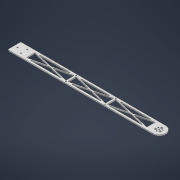
# Autodesk Inventor part: Top_Arm
Saved by Autodesk Inventor 2022 (Build 260153000, 153)
## iProperties
Created: 2023-02-15
Part Number: Top_Arm
Material: Generic
Document SubType Name: Modeling
Designer: dzw04
Density: 1 g/cm^3
Appearance: Default
Author: dzw04
Autodesk Inventor part; units mm, degrees
ref_plane "YZ Plane" through (0, 0, 0) normal (1, 0, 0) x (0, 1, 0)
ref_plane "XZ Plane" through (0, 0, 0) normal (0, 1, 0) x (-1, 0, 0)
ref_plane "XY Plane" through (0, 0, 0) normal (0, 0, 1) x (1, 0, 0)
sketch "Sketch1" plane through (0, 0, 0) normal (0, 1, 0) x (-1, 0, 0)
  arc A0 (74.0881, -0.9737) -> (74.0881, 0.9737) centre (73.8602, 0) ccw
  line L0 (74.0881, 0.9737) -> (26.2278, 12.1722)
  arc A1 (26.2278, 12.1722) -> (25, 11.1985) centre (26, 11.1985) ccw
  line L1 (25, 11.1985) -> (25, -11.1985)
  arc A2 (25, -11.1985) -> (26.2278, -12.1722) centre (26, -11.1985) ccw
  line L2 (26.2278, -12.1722) -> (74.0881, -0.9737)
  circle A3 centre (410, -10) radius 1.5
  line L3 (250.0605, -12.029) -> (212.2835, -2.7232)
  arc A4 (212.2835, -2.7232) -> (202.7161, -2.7232) centre (207.4998, -22.1427) ccw
  line L4 (202.7161, -2.7232) -> (164.9392, -12.029)
  arc A5 (164.9392, -12.029) -> (165.1783, -14) centre (165.1783, -13) ccw
  line L5 (165.1783, -14) -> (249.8213, -14)
  arc A6 (249.8213, -14) -> (250.0605, -12.029) centre (249.8213, -13) ccw
  line L6 (212.2835, 2.7232) -> (250.0605, 12.029)
  arc A7 (250.0605, 12.029) -> (249.8213, 14) centre (249.8213, 13) ccw
  line L7 (249.8213, 14) -> (165.1783, 14)
  arc A8 (165.1783, 14) -> (164.9392, 12.029) centre (165.1783, 13) ccw
  line L8 (164.9392, 12.029) -> (202.7161, 2.7232)
  arc A9 (202.7161, 2.7232) -> (212.2835, 2.7232) centre (207.4998, 22.1427) ccw
  circle A10 centre (6.4952, -3.75) radius 1.5
  line L9 (80.2767, -2.6067) -> (40.0191, -12.0263)
  arc A11 (40.0191, -12.0263) -> (40.2469, -14) centre (40.2469, -13) ccw
  line L10 (40.2469, -14) -> (129.4198, -14)
  arc A12 (129.4198, -14) -> (129.6476, -12.0263) centre (129.4198, -13) ccw
  line L11 (129.6476, -12.0263) -> (89.3899, -2.6067)
  arc A13 (89.3899, -2.6067) -> (80.2767, -2.6067) centre (84.8333, -22.0807) ccw
  line L12 (374.9809, -12.0263) -> (334.7231, -2.6067)
  arc A14 (334.7231, -2.6067) -> (325.6099, -2.6067) centre (330.1665, -22.0807) ccw
  line L13 (325.6099, -2.6067) -> (285.3521, -12.0263)
  arc A15 (285.3521, -12.0263) -> (285.58, -14) centre (285.58, -13) ccw
  line L14 (285.58, -14) -> (374.753, -14)
  arc A16 (374.753, -14) -> (374.9809, -12.0263) centre (374.753, -13) ccw
  line L15 (150.6667, 11.1789) -> (150.6667, -11.1789)
  arc A17 (150.6667, -11.1789) -> (151.9059, -12.1499) centre (151.6667, -11.1789) ccw
  line L16 (151.9059, -12.1499) -> (197.2869, -0.971)
  arc A18 (197.2869, -0.971) -> (197.2869, 0.971) centre (197.0477, 0) ccw
  line L17 (197.2869, 0.971) -> (151.9059, 12.1499)
  arc A19 (151.9059, 12.1499) -> (150.6667, 11.1789) centre (151.6667, 11.1789) ccw
  circle A20 centre (0, 0) radius 1.5
  circle A21 centre (6.4952, 3.75) radius 2.75
  line L18 (89.3899, 2.6067) -> (138.0828, 14)
  line L19 (138.0828, 14) -> (40.2469, 14)
  arc A22 (40.2469, 14) -> (40.0191, 12.0263) centre (40.2469, 13) ccw
  line L20 (40.0191, 12.0263) -> (80.2767, 2.6067)
  arc A23 (80.2767, 2.6067) -> (89.3899, 2.6067) centre (84.8333, 22.0807) ccw
  arc A24 (388.7722, -12.1722) -> (390, -11.1985) centre (389, -11.1985) ccw
  line L21 (390, -11.1985) -> (390, 11.1985)
  arc A25 (390, 11.1985) -> (388.7722, 12.1722) centre (389, 11.1985) ccw
  line L22 (388.7722, 12.1722) -> (340.9118, 0.9737)
  arc A26 (340.9118, 0.9737) -> (340.9118, -0.9737) centre (341.1396, 0) ccw
  line L23 (340.9118, -0.9737) -> (388.7722, -12.1722)
  line L24 (334.7231, 2.6067) -> (374.9809, 12.0263)
  arc A27 (374.9809, 12.0263) -> (374.753, 14) centre (374.753, 13) ccw
  line L25 (374.753, 14) -> (285.58, 14)
  arc A28 (285.58, 14) -> (285.3521, 12.0263) centre (285.58, 13) ccw
  line L26 (285.3521, 12.0263) -> (325.6099, 2.6067)
  arc A29 (325.6099, 2.6067) -> (334.7231, 2.6067) centre (330.1665, 22.0807) ccw
  circle A30 centre (430, 0) radius 1.5
  circle A31 centre (0, -7.5) radius 2.75
  circle A32 centre (0, 7.5) radius 1.5
  line L27 (144.6667, -11.1985) -> (144.6667, 11.1985)
  arc A33 (144.6667, 11.1985) -> (143.4388, 12.1722) centre (143.6667, 11.1985) ccw
  line L28 (143.4388, 12.1722) -> (95.5786, 0.9737)
  arc A34 (95.5786, 0.9737) -> (95.5786, -0.9737) centre (95.8064, 0) ccw
  line L29 (95.5786, -0.9737) -> (143.4388, -12.1722)
  arc A35 (143.4388, -12.1722) -> (144.6667, -11.1985) centre (143.6667, -11.1985) ccw
  arc A36 (264.333, 11.1789) -> (263.0938, 12.1499) centre (263.333, 11.1789) ccw
  line L30 (263.0938, 12.1499) -> (217.7128, 0.971)
  arc A37 (217.7128, 0.971) -> (217.7128, -0.971) centre (217.952, 0) ccw
  line L31 (217.7128, -0.971) -> (263.0938, -12.1499)
  arc A38 (263.0938, -12.1499) -> (264.333, -11.1789) centre (263.333, -11.1789) ccw
  line L32 (264.333, -11.1789) -> (264.333, 11.1789)
  circle A39 centre (410, 10) radius 1.5
  circle A40 centre (-6.4952, -3.75) radius 1.5
  circle A41 centre (-6.4952, 3.75) radius 2.75
  line L33 (271.5608, -12.1722) -> (319.4212, -0.9737)
  arc A42 (319.4212, -0.9737) -> (319.4212, 0.9737) centre (319.1934, 0) ccw
  line L34 (319.4212, 0.9737) -> (271.5608, 12.1722)
  arc A43 (271.5608, 12.1722) -> (270.333, 11.1985) centre (271.333, 11.1985) ccw
  line L35 (270.333, 11.1985) -> (270.333, -11.1985)
  arc A44 (270.333, -11.1985) -> (271.5608, -12.1722) centre (271.333, -11.1985) ccw
  arc A45 (440, 17.5) -> (437.5, 20) centre (437.5, 17.5) ccw
  line L36 (437.5, 20) -> (0, 20)
  arc A46 (0, 20) -> (0, -20) centre (0, 0) ccw
  line L37 (0, -20) -> (437.5, -20)
  arc A47 (437.5, -20) -> (440, -17.5) centre (437.5, -17.5) ccw
  line L38 (440, -17.5) -> (440, 17.5)
  point P0 (437.5, 20)
  point P1 (270.333, -11.1985)
  point P2 (270.333, 11.1985)
  point P3 (319.4212, 0.9737)
  point P4 (264.333, -11.1789)
  point P5 (217.7128, -0.971)
  point P6 (217.7128, 0.971)
  point P7 (263.0938, 12.1499)
  point P8 (95.5786, -0.9737)
  point P9 (325.6099, 2.6067)
  point P10 (285.3521, 12.0263)
  point P11 (374.753, 14)
  point P12 (340.9118, -0.9737)
  point P13 (388.7722, 12.1722)
  point P14 (390, 11.1985)
  point P15 (390, -11.1985)
  point P16 (80.2767, 2.6067)
  point P17 (40.0191, 12.0263)
  point P18 (197.2869, 0.971)
  point P19 (197.2869, -0.971)
  point P20 (325.6099, -2.6067)
  point P21 (334.7231, -2.6067)
  point P22 (129.6476, -12.0263)
  point P23 (164.9392, 12.029)
  point P24 (165.1783, -14)
  point P25 (202.7161, -2.7232)
  point P26 (212.2835, -2.7232)
  point P27 (74.0881, -0.9737)
  point P28 (25, 11.1985)
  point P29 (74.0881, 0.9737)
  constraints: 78 end point, 76 point on circle, 48 centre point
extrude "Extrusion1" add sketch "Sketch1" along normal blind 3
sketch "Sketch2" plane through (0, 3, 0) normal (0, 1, 0) x (1, 0, 0)
  line L0 (-144.6667, -11.1985) -> (-144.6667, 11.1985) construction
  line L1 (-144.6667, 0) -> (-150.6667, 0) construction
  line L2 (-150.6667, 11.1789) -> (-150.6667, -11.1789) construction
  line L3 (-264.333, -11.1789) -> (-264.333, 11.1789) construction
  line L4 (-264.333, 0) -> (-270.333, 0) construction
  line L5 (-270.333, 11.1985) -> (-270.333, -11.1985) construction
  line L6 (-147.6667, 0) -> (-147.6667, -15.75) construction
  line L7 (-437.5, -20) -> (0, -20) construction
  line L8 (-147.6667, 0) -> (-147.6667, 15.75) construction
  line L9 (-267.333, 0) -> (-267.333, -15.75) construction
  line L10 (-267.333, 0) -> (-267.333, 15.75) construction
  circle A0 centre (-147.6667, -15.75) radius 1.5
  circle A1 centre (-147.6667, 15.75) radius 1.5
  circle A2 centre (-267.333, -15.75) radius 1.5
  circle A3 centre (-267.333, 15.75) radius 1.5
  point P0 (0, 0)
  dimension "d2" = 15.75
  dimension "d3" = 15.75
  dimension "d4" = 15.75
  dimension "d5" = 3
  dimension "d6" = 3
  dimension "d7" = 3
  dimension "d8" = 3
  constraints: 12 end point, 6 midpoint, 4 centre point, 4 coincident, 3 vertical, 1 perpendicular
  measures "d2" distance of L6.start L6.end
  measures "d3" distance of L6.start L8.end
  measures "d4" distance of L9.start L9.end
  measures "d5" diameter of A0
  measures "d6" diameter of A1
  measures "d7" diameter of A2
  measures "d8" diameter of A3
extrude "Extrusion2" cut sketch "Sketch2" against normal blind 3
equation "\"d9\" = d5"
body "Solid1"
